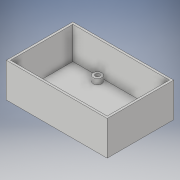
# Autodesk Inventor part: MainPCB_RPI_Case
Saved by Autodesk Inventor 2019.4 (Build 234330000, 330)
## iProperties
Created: 2020-03-12
Part Number: MainPCB_RPI_Case
Material: Generic
Document SubType Name: Modeling
Designer: Jorian Bruslind
Density: 1 g/cm^3
Appearance: Default
Author: Jorian Bruslind
Autodesk Inventor part; units mm, degrees
ref_plane "YZ Plane" through (0, 0, 0) normal (1, 0, 0) x (0, 1, 0)
ref_plane "XZ Plane" through (0, 0, 0) normal (0, 1, 0) x (-1, 0, 0)
ref_plane "XY Plane" through (0, 0, 0) normal (0, 0, 1) x (1, 0, 0)
sketch "Sketch1" plane through (0, 0, 0) normal (0, 1, 0) x (-1, 0, 0)
  line L0 (0, 0) -> (90, 0)
  line L1 (90, 0) -> (90, -58)
  line L2 (90, -58) -> (0, -58)
  line L3 (0, -58) -> (0, 0)
  line L4 (92, -60) -> (92, 2)
  line L5 (92, 2) -> (-2, 2)
  line L6 (-2, 2) -> (-2, -60)
  line L7 (-2, -60) -> (92, -60)
  dimension "d0" = 90
  dimension "d1" = 58
  dimension "d2" = 2
  constraints: 16 end point, 4 parallel, 2 perpendicular, 1 horizontal, 3 other
  measures "d0" distance of L1.end L2.end
  measures "d1" distance of L0.end L1.end
  measures "d2" distance between parallel lines of L1 L4
extrude "Extrusion1" add sketch "Sketch1" along normal blind 32 contours L0 L1 L2 L3 | L7 L6 L5 L4
sketch "Sketch2" plane through (0, 32, 0) normal (0, 1, 0) x (1, 0, 0)
  line L0 (0, 0) -> (-90, 0)
  line L1 (-90, 0) -> (-90, 58)
  line L2 (-90, 58) -> (0, 58)
  line L3 (0, 58) -> (0, 0)
  dimension "d5" = 90
  dimension "d6" = 58
  constraints: 8 end point, 2 parallel, 1 horizontal, 1 perpendicular
  measures "d5" distance of L1.end L2.end
  measures "d6" distance of L0.end L1.end
extrude "Extrusion2" cut sketch "Sketch2" against normal blind 30
sketch "Sketch3" plane through (0, 2, 0) normal (0, 1, 0) x (1, 0, 0)
  line L0 (0, 58) -> (0, 0) projected
  line L1 (0, 0) -> (0, 4.5)
  line L2 (0, 4.5) -> (-4.5, 4.5)
  circle A0 centre (-4.5, 4.5) radius 2
  circle A1 centre (-4.5, 4.5) radius 4
  circle A2 centre (-4.5, 53.5) radius 4
  circle A3 centre (-4.5, 53.5) radius 2
  circle A4 centre (-62.5, 4.5) radius 4
  circle A5 centre (-62.5, 4.5) radius 2
  circle A6 centre (-62.5, 53.5) radius 4
  circle A7 centre (-62.5, 53.5) radius 2
  dimension "d9" = 4.5
  dimension "d10" = 4.5
  dimension "d11" = 4
  dimension "d12" = 8
  dimension "d15" = 49
  dimension "d18" = 58
  constraints: 8 centre point, 5 coincident, 4 end point, 1 horizontal, 1 perpendicular, 1 point on line, 1 vertical, 12 other
  measures "d9" distance of L0.end L1.end
  measures "d10" distance of L1.end L2.end
  measures "d11" diameter of A0
  measures "d12" diameter of A1
  measures "d15" distance of A1.centre A2.centre
  measures "d18" distance of A1.centre A4.centre
extrude "Extrusion3" add sketch "Sketch3" along normal blind 5
body "Solid1"
